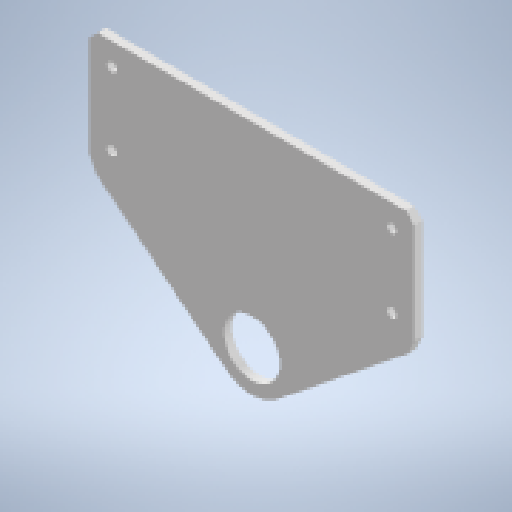
# Autodesk Inventor part: A_B_hinge
Saved by Autodesk Inventor 2025.2 (Build 292293000, 293)
## iProperties
Created: 2025-04-08
Part Number: A_B_hinge
Material: Generic
Document SubType Name: Sheet Metal
Designer: Caspe
Density: 1 g/cm^3
Sheet Metal Rule: Default_mm
Appearance: Default
Flat Pattern Width: 8.45 cm
Flat Pattern Length: 11.6 cm
Flat Pattern Area: 98.02 cm^2
Sheet Metal Width: 84,500 mm
Sheet Metal Length: 116,000 mm
Sheet Metal Area: 9802,000 mm^2
Mass: 21.5483 g
Surface Area: 157.016 cm^2
Volume: 21.5483 cm^3
Author: Caspe
Autodesk Inventor part; units mm, degrees
ref_plane "YZ Plane" through (0, 0, 0) normal (1, 0, 0) x (0, 1, 0)
ref_plane "XZ Plane" through (0, 0, 0) normal (0, 1, 0) x (-1, 0, 0)
ref_plane "XY Plane" through (0, 0, 0) normal (0, 0, 1) x (1, 0, 0)
sketch "Sketch1" plane through (0, 0, 0) normal (0, 0, 1) x (1, 0, 0)
  line L0 (0, 0) -> (116, 0)
  line L1 (116, 0) -> (116, -42)
  line L2 (0, 0) -> (0, -42)
  circle A0 centre (8, -8) radius 1.675
  circle A1 centre (108, -8) radius 1.675
  circle A2 centre (8, -34) radius 1.675
  circle A3 centre (108, -34) radius 1.675
  circle A4 centre (58, -70) radius 10
  circle A5 centre (58, -70) radius 14.5
  line L3 (0, -42) -> (48.9181, -81.3035)
  line L4 (116, -42) -> (67.0819, -81.3035)
  dimension "d0" = 116
  dimension "d1" = 42
  dimension "d2" = 3.35
  dimension "d3" = 8
  dimension "d4" = 8
  dimension "d7" = 100
  dimension "d10" = 26
  dimension "d13" = 42
  dimension "d14" = 20
  dimension "d15" = 29
  dimension "d16" = 70
  measures "d0" distance of L0.start L0.end
  measures "d1" distance of L0.end L1.end
  measures "d2" diameter of A0
  measures "d3" distance from line of L0 A0.centre
  measures "d4" distance from line of L2 A0.centre
  measures "d7" distance of A0.centre A1.centre
  measures "d10" distance of A0.centre A2.centre
  measures "d13" distance of L0.start L2.end
  measures "d14" diameter of A4
  measures "d15" diameter of A5
  measures "d16" distance from line of L0 A4.centre
extrude "Plate1" add sketch "Sketch1" along normal blind 3
chamfer "Corner Chamfer1" distance 3 angle 45 4 edges at (0, -42, 1.5) (0, 0, 1.5) (116, 0, 1.5) (116, -42, 1.5)
equation "\"d2\" = rivet_diameter"
equation "\"d13\" = d1"
equation "\"d17\" = Thickness"
equation "\"BendRadius\" = Thickness"
equation "\"BendReliefWidth\" = Thickness"
equation "\"BendReliefDepth\" = 0.5 * Thickness"
equation "\"CornerReliefSize\" = 4 * Thickness"
equation "\"MinimumRemnant\" = 2 * Thickness"
equation "\"TransitionRadius\" = BendRadius"
equation "\"JacobiRadiusSize\" = BendRadius"
equation "\"GapSize\" = Thickness"
equation "\"A_width\" = 46"
equation "\"A_joint_diameter\" = 16"
equation "\"A_joint_tolerance\" = 3"
equation "\"l___________\" = 0"
equation "\"l__________\" = 0"
equation "\"l_________\" = 0"
equation "\"rivet_diameter\" = 3.35"
equation "\"plate_thickness\" = 3"
equation "\"l________\" = 0"
equation "\"A_B_spacing\" = 2"
equation "\"L_Piston_Bottom\" = 21"
equation "\"L_Piston_Top\" = 25"
equation "\"thin_plate\" = 1.5"
equation "\"Thickness\" = 3"
body "Solid1"
